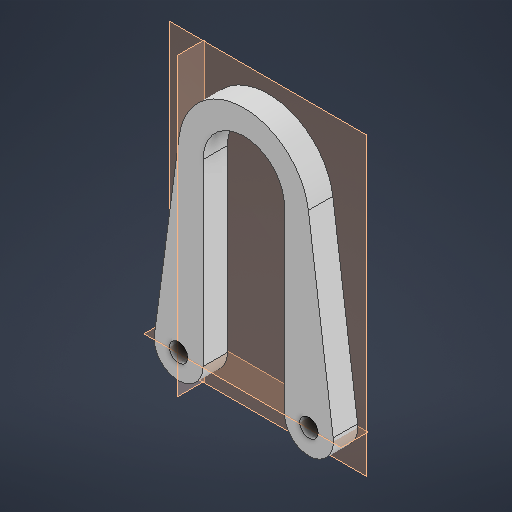
# Autodesk Inventor part: gpu_cable_holder
Saved by Autodesk Inventor 2026.2 (Build 302298010, 298A)
## iProperties
Created: 2026-03-06
Part Number: gpu_cable_holder
Material: Generic
Document SubType Name: Modeling
Designer: numai
Density: 1 g/cm^3
Appearance: Default
Author: numai
Autodesk Inventor part; units mm, degrees
sketch "スケッチ1" plane through (0, 0, 0) normal (0, 0, 1) x (1, 0, 0)
  line L0 (0, 0) -> (32, 0) construction
  line L1 (0, 60) -> (36, 60) construction
  circle A0 centre (0, 0) radius 2.25
  circle A1 centre (32, 0) radius 2.25
  circle A2 centre (16, 44) radius 10
  circle A3 centre (0, 0) radius 6
  circle A4 centre (32, 0) radius 6
  line L2 (6, 44) -> (6, 0)
  line L3 (26, 44) -> (26, 0)
  line L4 (-5.9466, 0.7988) -> (0.1424, 46.13)
  arc A5 (31.8576, 46.13) -> (0.1424, 46.13) centre (16, 44) ccw
  line L5 (31.8576, 46.13) -> (37.9466, 0.7988)
  point P0 (16, 0)
  dimension "d4" = 4.5
  dimension "d11" = 32
  dimension "d12" = 12
  dimension "d14" = 60
  dimension "d15" = 20
  dimension "d16" = 6
  constraints: 12 end point, 9 tangent, 8 point on circle, 6 centre point, 5 coincident, 3 vertical alignment, 2 equal radius, 2 horizontal, 1 concentric, 1 midpoint
  measures "d4" diameter of A0
  measures "d11" distance of L0.end L0.start
  measures "d12" diameter of A3
  measures "d14" distance between parallel lines of L0 L1
  measures "d15" diameter of A2
  measures "d16" radial gap between concentric circles of A5 A2
extrude "押し出し1" add sketch "スケッチ1" along normal blind 6 contours A2 L2 A3 L4 A5 L5 A4 L3 | A4 | A3
sketch "スケッチ4" plane through (0, 0, 0) normal (0, 0, -1) x (-1, 0, 0)
  circle A0 centre (-32, 0) radius 2.25 construction
  circle A1 centre (0, 0) radius 2.25 construction
  circle A2 centre (-32, 0) radius 4
  circle A3 centre (0, 0) radius 4
  dimension "d17" = 8
  constraints: 2 centre point, 2 coincident, 1 equal radius
  measures "d17" diameter of A2
extrude "押し出し3" cut sketch "スケッチ4" against normal blind 2
